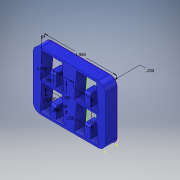
# Autodesk Inventor part: AW5.5bPassenger Base
Saved by Autodesk Inventor 2018 (Build 220112000, 112)
## iProperties
Created: 2019-01-22
Part Number: AW5.5bPassenger Base
Material: Generic
Document SubType Name: Modeling
Designer: russd
Density: 1 g/cm^3
Appearance: Blue - Wall Paint - Glossy
Author: russd
Autodesk Inventor part; units mm, degrees
ref_plane "YZ Plane" through (0, 0, 0) normal (1, 0, 0) x (0, 1, 0)
ref_plane "XZ Plane" through (0, 0, 0) normal (0, 1, 0) x (-1, 0, 0)
ref_plane "XY Plane" through (0, 0, 0) normal (0, 0, 1) x (1, 0, 0)
sketch "Sketch1" plane through (0, 0, 0) normal (0, 0, 1) x (1, 0, 0)
  line L0 (-5.08, 0) -> (-45.212, 0)
  line L1 (-50.292, 5.08) -> (-50.292, 35.306)
  line L2 (-45.212, 40.386) -> (-5.08, 40.386)
  line L3 (0, 35.306) -> (0, 5.08)
  line L4 (-45.466, 1.524) -> (-43.942, 19.558)
  line L5 (-43.942, 19.558) -> (-30.226, 19.558)
  line L6 (-30.226, 19.558) -> (-28.702, 1.524)
  line L7 (-28.702, 1.524) -> (-35.052, 1.524)
  line L8 (-35.052, 1.524) -> (-35.052, 9.652)
  line L9 (-35.052, 9.652) -> (-39.116, 9.652)
  line L10 (-39.116, 9.652) -> (-39.116, 1.524)
  line L11 (-39.116, 1.524) -> (-45.466, 1.524)
  line L12 (-35.052, 20.828) -> (-35.052, 28.956)
  line L13 (-35.052, 28.956) -> (-39.116, 28.956)
  line L14 (-43.942, 38.862) -> (-30.226, 38.862)
  line L15 (-28.702, 20.828) -> (-35.052, 20.828)
  line L16 (-30.226, 38.862) -> (-28.702, 20.828)
  line L17 (-39.116, 28.956) -> (-39.116, 20.828)
  line L18 (-39.116, 20.828) -> (-45.466, 20.828)
  line L19 (-45.466, 20.828) -> (-43.942, 38.862)
  line L20 (-4.826, 1.524) -> (-6.35, 19.558)
  line L21 (-6.35, 19.558) -> (-20.066, 19.558)
  line L22 (-20.066, 19.558) -> (-21.59, 1.524)
  line L23 (-21.59, 1.524) -> (-15.24, 1.524)
  line L24 (-15.24, 1.524) -> (-15.24, 9.652)
  line L25 (-15.24, 9.652) -> (-11.176, 9.652)
  line L26 (-11.176, 9.652) -> (-11.176, 1.524)
  line L27 (-11.176, 1.524) -> (-4.826, 1.524)
  line L28 (-15.24, 20.828) -> (-15.24, 28.956)
  line L29 (-15.24, 28.956) -> (-11.176, 28.956)
  line L30 (-6.35, 38.862) -> (-20.066, 38.862)
  line L31 (-21.59, 20.828) -> (-15.24, 20.828)
  line L32 (-20.066, 38.862) -> (-21.59, 20.828)
  line L33 (-11.176, 28.956) -> (-11.176, 20.828)
  line L34 (-11.176, 20.828) -> (-4.826, 20.828)
  line L35 (-4.826, 20.828) -> (-6.35, 38.862)
  arc A0 (0, 35.306) -> (-5.08, 40.386) centre (-5.08, 35.306) ccw
  arc A1 (-45.212, 40.386) -> (-50.292, 35.306) centre (-45.212, 35.306) ccw
  arc A2 (-50.292, 5.08) -> (-45.212, 0) centre (-45.212, 5.08) ccw
  arc A3 (-5.08, 0) -> (0, 5.08) centre (-5.08, 5.08) ccw
  point P0 (0, 0)
  point P1 (-50.292, 40.386)
  point P2 (-50.292, 0)
  point P3 (0, 40.386)
  dimension "d0" = 50.292
  dimension "d1" = 40.386
  dimension "d2" = 4.826
  dimension "d3" = 6.35
  dimension "d4" = 6.35
  dimension "d6" = 13.716
  dimension "d7" = 6.35
  dimension "d8" = 1.524
  dimension "d10" = 8.128
  dimension "d12" = 4.064
  dimension "d13" = 18.034
  dimension "d16" = 19.304
  dimension "d21" = 5.08
  constraints: 72 end point, 12 point on line, 8 point on circle, 8 tangent, 5 perpendicular, 4 centre point, 3 equal radius, 3 parallel, 2 horizontal, 1 vertical, 16 other
  measures "d0" distance of point (-50.292, 40.386) point (0, 40.386)
  measures "d1" distance of point (-50.292, 0) point (-50.292, 40.386)
  measures "d2" distance from line of L4.start L1
  measures "d3" distance of L10.end L4.start
  measures "d4" distance of L6.end L7.end
  measures "d6" distance of L4.end L5.end
  measures "d7" distance from line of L1 L4.end
  measures "d8" distance between parallel lines of L11 L0
  measures "d10" distance between parallel lines of L9 L11
  measures "d12" distance between parallel lines of L8 L10
  measures "d13" distance between parallel lines of L7 L5
  measures "d16" distance of L7.end L12.start
  measures "d21" radius of A0
extrude "Extrusion1" add sketch "Sketch1" along normal blind 7.874
sketch "Sketch2" plane through (0, 0, 7.874) normal (0, 0, 1) x (1, 0, 0)
  point P0 (0, 0)
sketch "Sketch3" plane through (0, 0, 7.874) normal (0, 0, 1) x (1, 0, 0)
  line L0 (-4.826, 20.828) -> (-11.176, 20.828) projected
  line L1 (-11.176, 20.828) -> (-11.176, 28.956) projected
  line L2 (-11.176, 28.956) -> (-15.24, 28.956) projected
  line L3 (-15.24, 28.956) -> (-15.24, 20.828) projected
  line L4 (-15.24, 20.828) -> (-21.59, 20.828) projected
  line L5 (-21.59, 20.828) -> (-20.066, 38.862) projected
  line L6 (-20.066, 38.862) -> (-6.35, 38.862) projected
  line L7 (-6.35, 38.862) -> (-4.826, 20.828) projected
  line L8 (-4.826, 1.524) -> (-11.176, 1.524) projected
  line L9 (-11.176, 1.524) -> (-11.176, 9.652) projected
  line L10 (-11.176, 9.652) -> (-15.24, 9.652) projected
  line L11 (-15.24, 9.652) -> (-15.24, 1.524) projected
  line L12 (-15.24, 1.524) -> (-21.59, 1.524) projected
  line L13 (-21.59, 1.524) -> (-20.066, 19.558) projected
  line L14 (-20.066, 19.558) -> (-6.35, 19.558) projected
  line L15 (-6.35, 19.558) -> (-4.826, 1.524) projected
  line L16 (-35.052, 20.828) -> (-35.052, 28.956) projected
  line L17 (-35.052, 28.956) -> (-39.116, 28.956) projected
  line L18 (-39.116, 28.956) -> (-39.116, 20.828) projected
  line L19 (-39.116, 20.828) -> (-45.466, 20.828) projected
  line L20 (-45.466, 20.828) -> (-43.942, 38.862) projected
  line L21 (-43.942, 38.862) -> (-30.226, 38.862) projected
  line L22 (-30.226, 38.862) -> (-28.702, 20.828) projected
  line L23 (-28.702, 20.828) -> (-35.052, 20.828) projected
  line L24 (-43.942, 19.558) -> (-30.226, 19.558) projected
  line L25 (-30.226, 19.558) -> (-28.702, 1.524) projected
  line L26 (-28.702, 1.524) -> (-35.052, 1.524) projected
  line L27 (-35.052, 1.524) -> (-35.052, 9.652) projected
  line L28 (-35.052, 9.652) -> (-39.116, 9.652) projected
  line L29 (-39.116, 9.652) -> (-39.116, 1.524) projected
  line L30 (-39.116, 1.524) -> (-45.466, 1.524) projected
  line L31 (-45.466, 1.524) -> (-43.942, 19.558) projected
  line L32 (-5.08, 40.386) -> (-45.212, 40.386) projected
  arc A0 (-45.212, 40.386) -> (-50.292, 35.306) centre (-45.212, 35.306) ccw projected
  line L33 (-50.292, 35.306) -> (-50.292, 5.08) projected
  arc A1 (-50.292, 5.08) -> (-45.212, 0) centre (-45.212, 5.08) ccw projected
  line L34 (-45.212, 0) -> (-5.08, 0) projected
  arc A2 (-5.08, 0) -> (0, 5.08) centre (-5.08, 5.08) ccw projected
  line L35 (0, 5.08) -> (0, 35.306) projected
  arc A3 (0, 35.306) -> (-5.08, 40.386) centre (-5.08, 35.306) ccw projected
  line L36 (-39.116, 20.828) -> (-39.116, 28.956) projected
  line L37 (-35.052, 28.956) -> (-35.052, 20.828) projected
  line L38 (-39.116, 28.956) -> (-35.052, 28.956)
  line L39 (-35.052, 28.956) -> (-35.052, 20.828)
  line L40 (-35.052, 20.828) -> (-39.116, 20.828)
  line L41 (-39.116, 20.828) -> (-39.116, 28.956)
  line L42 (-15.24, 28.956) -> (-15.24, 20.828) projected
  line L43 (-11.176, 20.828) -> (-11.176, 28.956) projected
  line L44 (-15.24, 28.956) -> (-11.176, 28.956)
  line L45 (-11.176, 28.956) -> (-11.176, 20.828)
  line L46 (-11.176, 20.828) -> (-15.24, 20.828)
  line L47 (-15.24, 20.828) -> (-15.24, 28.956)
  line L48 (-15.24, 9.652) -> (-15.24, 1.524) projected
  line L49 (-11.176, 1.524) -> (-15.24, 1.524)
  line L50 (-15.24, 1.524) -> (-15.24, 9.652)
  line L51 (-15.24, 9.652) -> (-11.176, 9.652)
  line L52 (-11.176, 9.652) -> (-11.176, 1.524)
  line L53 (-35.052, 9.652) -> (-39.116, 9.652) projected
  line L54 (-35.052, 1.524) -> (-28.702, 1.524) projected
  line L55 (-39.116, 9.652) -> (-35.052, 9.652)
  line L56 (-35.052, 9.652) -> (-35.052, 1.524)
  line L57 (-35.052, 1.524) -> (-39.116, 1.524)
  line L58 (-39.116, 1.524) -> (-39.116, 9.652)
  point P0 (0, 0)
  constraints: 32 end point, 8 parallel, 4 horizontal, 4 perpendicular
extrude "Extrusion2" cut sketch "Sketch3" against normal blind 0.762 contours L46 L3 L2 L1 | L49 L11 L10 L9 | L40 L18 L17 L16 | L29 L28 L27 L57
fillet "Fillet1" radius 1.27 4 edges at (-37.084, 28.956, 7.112) (-13.208, 28.956, 7.112) (-37.084, 9.652, 7.112) (-13.208, 9.652, 7.112)
shell "Shell1" thickness 0.254 removed faces 1 at (-26.3313, 32.8507, 0)
body "Solid1"
